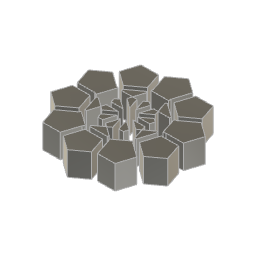
_Vent Pattern.50e8ad99-56d1-49d6-96c2-bcab84f8e137 (Autodesk Fusion 360 design; units mm, degrees)
Autodesk Fusion 360 part; units mm, degrees
note: some values were not read from the file. Chosen so that the rebuilt part matches the saved one: which bodies a step acts on.
sketch "Sketch1" plane through (0, 0, 16.5) normal (0, 0, 1) x (-1, 0, 0)
  line L0 (-58.1352, 10.5579) -> (-59.2385, 7.0968)
  line L1 (-59.2385, 7.0968) -> (-56.2877, 4.9779)
  line L2 (-56.2877, 4.9779) -> (-53.3607, 7.1296)
  line L3 (-53.3607, 7.1296) -> (-54.5025, 10.5782)
  line L4 (-54.5025, 10.5782) -> (-58.1352, 10.5579)
  line L5 (-54.5025, 10.5782) -> (-53.3607, 7.1296)
  line L6 (-53.3607, 7.1296) -> (-52.8861, 7.2867)
  line L7 (-52.8861, 7.2867) -> (-54.0279, 10.7353)
  line L8 (-54.0279, 10.7353) -> (-54.5025, 10.5782)
  line L9 (-58.1352, 10.5579) -> (-59.2385, 7.0968)
  line L10 (-59.2385, 7.0968) -> (-59.7149, 7.2486)
  line L11 (-59.7149, 7.2486) -> (-58.6116, 10.7098)
  line L12 (-58.6116, 10.7098) -> (-58.1352, 10.5579)
  line L13 (-50.6262, 13.0441) -> (-47.6754, 10.9252)
  line L14 (-47.3838, 11.3314) -> (-50.3346, 13.4502)
  line L15 (-48.7787, 7.4641) -> (-52.4114, 7.4439)
  line L16 (-54.0279, 10.7353) -> (-53.5532, 10.8925)
  line L17 (-53.5532, 10.8925) -> (-50.6262, 13.0441)
  line L18 (-53.5532, 10.8925) -> (-52.4114, 7.4439)
  line L19 (-50.6262, 13.0441) -> (-47.6754, 10.9252)
  line L20 (-52.4114, 7.4439) -> (-52.8861, 7.2867)
  line L21 (-52.8861, 7.2867) -> (-54.0279, 10.7353)
  line L22 (-50.3346, 13.4502) -> (-50.6262, 13.0441)
  line L23 (-47.6754, 10.9252) -> (-48.7787, 7.4641)
  line L24 (-47.6754, 10.9252) -> (-47.3838, 11.3314)
  line L25 (-52.4114, 7.4439) -> (-53.5532, 10.8925)
  line L26 (-45.3098, 17.8377) -> (-48.9424, 17.8175)
  line L27 (-50.043, 13.8564) -> (-47.0922, 11.7375)
  line L28 (-48.9452, 18.3175) -> (-45.3126, 18.3377)
  line L29 (-47.3838, 11.3314) -> (-50.3346, 13.4502)
  line L30 (-45.307, 17.3377) -> (-48.9397, 17.3175)
  line L31 (-50.3346, 13.4502) -> (-50.043, 13.8564)
  line L32 (-47.0922, 11.7375) -> (-47.3838, 11.3314)
  line L33 (-48.9397, 17.3175) -> (-50.043, 13.8564)
  line L34 (-48.9424, 17.8175) -> (-48.9397, 17.3175)
  line L35 (-47.1601, 23.9177) -> (-47.4562, 24.3205)
  line L36 (-50.043, 13.8564) -> (-47.0922, 11.7375)
  line L37 (-45.3098, 17.8377) -> (-48.9424, 17.8175)
  line L38 (-48.9397, 17.3175) -> (-45.307, 17.3377)
  line L39 (-45.307, 17.3377) -> (-45.3098, 17.8377)
  line L40 (-44.1652, 13.8891) -> (-45.307, 17.3377)
  line L41 (-48.9424, 17.8175) -> (-48.9452, 18.3175)
  line L42 (-47.0922, 11.7375) -> (-44.1652, 13.8891)
  line L43 (-45.3126, 18.3377) -> (-45.3098, 17.8377)
  line L44 (-54.5025, 10.5782) -> (-58.1352, 10.5579)
  line L45 (-58.1352, 10.5579) -> (-58.138, 11.0579)
  line L46 (-58.138, 11.0579) -> (-54.5053, 11.0781)
  line L47 (-54.5053, 11.0781) -> (-54.5025, 10.5782)
  line L48 (-48.9397, 17.3175) -> (-50.043, 13.8564)
  line L49 (-50.043, 13.8564) -> (-50.5193, 14.0082)
  line L50 (-50.5193, 14.0082) -> (-49.416, 17.4693)
  line L51 (-49.416, 17.4693) -> (-48.9397, 17.3175)
  line L52 (-54.5081, 11.5781) -> (-58.1407, 11.5579)
  line L53 (-58.1407, 11.5579) -> (-59.2826, 15.0065)
  line L54 (-59.2826, 15.0065) -> (-56.3556, 17.1581)
  line L55 (-56.3556, 17.1581) -> (-53.4048, 15.0393)
  line L56 (-53.4048, 15.0393) -> (-54.5081, 11.5781)
  line L57 (-52.8432, 19.74) -> (-49.8924, 17.6212)
  line L58 (-55.7702, 17.5884) -> (-52.8432, 19.74)
  line L59 (-54.6284, 14.1398) -> (-55.7702, 17.5884)
  line L60 (-50.9957, 14.1601) -> (-54.6284, 14.1398)
  line L61 (-49.8924, 17.6212) -> (-50.9957, 14.1601)
  line L62 (-50.5193, 14.0082) -> (-49.416, 17.4693)
  line L63 (-58.2127, 24.4741) -> (-54.5801, 24.4943)
  line L64 (-53.4796, 28.4555) -> (-54.5829, 24.9943)
  line L65 (-54.1065, 24.8425) -> (-54.5829, 24.9943)
  line L66 (-58.2155, 24.9741) -> (-59.3573, 28.4227)
  line L67 (-53.4796, 28.4555) -> (-53.0032, 28.3036)
  line L68 (-59.832, 28.2655) -> (-58.6902, 24.8169)
  line L69 (-54.5829, 24.9943) -> (-58.2155, 24.9741)
  line L70 (-52.5268, 28.1517) -> (-53.0032, 28.3036)
  line L71 (-51.0364, 21.4517) -> (-54.669, 21.4315)
  line L72 (-53.6301, 24.6906) -> (-50.6793, 22.5718)
  line L73 (-54.5801, 24.4943) -> (-54.5829, 24.9943)
  line L74 (-54.669, 21.4315) -> (-55.7723, 17.9704)
  line L75 (-59.3573, 28.4227) -> (-59.832, 28.2655)
  line L76 (-53.0032, 28.3036) -> (-54.1065, 24.8425)
  line L77 (-54.5829, 24.9943) -> (-53.4796, 28.4555)
  line L78 (-56.3625, 18.3941) -> (-53.4355, 20.5458)
  line L79 (-58.21, 23.9741) -> (-59.3133, 20.513)
  line L80 (-48.8942, 28.172) -> (-52.5268, 28.1517)
  line L81 (-58.6902, 24.8169) -> (-58.2155, 24.9741)
  line L82 (-53.6301, 24.6906) -> (-52.5268, 28.1517)
  line L83 (-52.5268, 28.1517) -> (-53.6301, 24.6906)
  line L84 (-58.2155, 24.9741) -> (-59.3573, 28.4227)
  line L85 (-53.4355, 20.5458) -> (-54.5773, 23.9944)
  line L86 (-58.2155, 24.9741) -> (-58.2127, 24.4741)
  line L87 (-53.0032, 28.3036) -> (-54.1065, 24.8425)
  line L88 (-54.1065, 24.8425) -> (-53.6301, 24.6906)
  line L89 (-54.5773, 23.9944) -> (-58.21, 23.9741)
  line L90 (-49.4199, 18.1603) -> (-48.9452, 18.3175)
  line L91 (-47.1601, 23.9177) -> (-44.2093, 21.7988)
  line L92 (-48.9424, 17.8175) -> (-48.9397, 17.3175)
  line L93 (-45.3098, 17.8377) -> (-48.9424, 17.8175)
  line L94 (-45.3126, 18.3377) -> (-48.9452, 18.3175)
  line L95 (-54.5829, 24.9943) -> (-58.2155, 24.9741)
  line L96 (-45.307, 17.3377) -> (-45.3098, 17.8377)
  line L97 (-48.9452, 18.3175) -> (-45.3126, 18.3377)
  line L98 (-48.9452, 18.3175) -> (-50.087, 21.7661)
  line L99 (-47.7523, 24.7234) -> (-48.8942, 28.172)
  line L100 (-50.3832, 22.1689) -> (-50.087, 21.7661)
  line L101 (-48.9397, 17.3175) -> (-45.307, 17.3377)
  line L102 (-59.3133, 20.513) -> (-56.3625, 18.3941)
  line L103 (-47.4562, 24.3205) -> (-50.3832, 22.1689)
  line L104 (-45.3098, 17.8377) -> (-48.9424, 17.8175)
  line L105 (-49.8946, 18.0031) -> (-51.0364, 21.4517)
  line L106 (-48.9452, 18.3175) -> (-50.087, 21.7661)
  line L107 (-56.4304, 30.5743) -> (-53.4796, 28.4555)
  line L108 (-50.6793, 22.5718) -> (-47.7523, 24.7234)
  line L109 (-47.4562, 24.3205) -> (-50.3832, 22.1689)
  line L110 (-50.5617, 21.6089) -> (-49.4199, 18.1603)
  line L111 (-47.1601, 23.9177) -> (-47.4562, 24.3205)
  line L112 (-50.087, 21.7661) -> (-47.1601, 23.9177)
  line L113 (-50.5617, 21.6089) -> (-49.4199, 18.1603)
  line L114 (-50.087, 21.7661) -> (-50.5617, 21.6089)
  line L115 (-50.087, 21.7661) -> (-47.1601, 23.9177)
  line L116 (-47.7523, 24.7234) -> (-47.4562, 24.3205)
  line L117 (-50.3832, 22.1689) -> (-50.6793, 22.5718)
  line L118 (-52.8215, 15.8515) -> (-49.8946, 18.0031)
  line L119 (-44.2093, 21.7988) -> (-45.3126, 18.3377)
  line L120 (-59.3573, 28.4227) -> (-56.4304, 30.5743)
  line L121 (-48.9424, 17.8175) -> (-48.9452, 18.3175)
  line L122 (-50.6793, 22.5718) -> (-47.7523, 24.7234)
  line L123 (-55.7723, 17.9704) -> (-52.8215, 15.8515)
  line L124 (-45.3126, 18.3377) -> (-45.3098, 17.8377)
  line L125 (-57.0963, 13.817) -> (-54.1455, 11.6982)
  line L126 (-53.8493, 11.2953) -> (-53.5532, 10.8925)
  line L127 (-52.3603, 17.2984) -> (-55.993, 17.2782)
  line L128 (-52.4114, 7.4439) -> (-52.8861, 7.2867)
  line L129 (-68.5088, 13.7534) -> (-65.558, 11.6346)
  line L130 (-51.2185, 13.8498) -> (-52.3603, 17.2984)
  line L131 (-53.5532, 10.8925) -> (-52.4114, 7.4439)
  line L132 (-67.4055, 17.2145) -> (-67.4083, 17.7145)
  line L133 (-67.4055, 17.2145) -> (-68.5088, 13.7534)
  line L134 (-47.3838, 11.3314) -> (-50.3346, 13.4502)
  line L135 (-50.6262, 13.0441) -> (-47.6754, 10.9252)
  line L136 (-53.5532, 10.8925) -> (-50.6262, 13.0441)
  line L137 (-54.5025, 10.5782) -> (-58.1352, 10.5579)
  line L138 (-50.3346, 13.4502) -> (-50.6262, 13.0441)
  line L139 (-65.558, 11.6346) -> (-65.2618, 11.2317)
  line L140 (-56.2877, 4.9779) -> (-53.3607, 7.1296)
  line L141 (-47.6754, 10.9252) -> (-47.3838, 11.3314)
  line L142 (-54.1455, 11.6982) -> (-51.2185, 13.8498)
  line L143 (-67.4055, 17.2145) -> (-67.4083, 17.7145)
  line L144 (-63.7728, 17.2348) -> (-63.2982, 17.392)
  line L145 (-62.631, 13.7862) -> (-63.7728, 17.2348)
  line L146 (-53.5532, 10.8925) -> (-50.6262, 13.0441)
  line L147 (-65.558, 11.6346) -> (-65.2618, 11.2317)
  line L148 (-58.5047, 11.6739) -> (-55.5777, 13.8255)
  line L149 (-50.6262, 13.0441) -> (-50.9224, 13.4469)
  line L150 (-50.6262, 13.0441) -> (-47.6754, 10.9252)
  line L151 (-50.9224, 13.4469) -> (-53.8493, 11.2953)
  line L152 (-62.0387, 12.9805) -> (-64.9657, 10.8289)
  line L153 (-58.7963, 11.2678) -> (-61.7471, 13.3866)
  line L154 (-54.0279, 10.7353) -> (-54.5025, 10.5782)
  line L155 (-54.0279, 10.7353) -> (-53.5532, 10.8925)
  line L156 (-59.2385, 7.0968) -> (-59.7149, 7.2486)
  line L157 (-55.5777, 13.8255) -> (-56.7195, 17.2741)
  line L158 (-59.0879, 10.8616) -> (-60.1912, 7.4005)
  line L159 (-60.1912, 7.4005) -> (-59.7149, 7.2486)
  line L160 (-53.3607, 7.1296) -> (-52.8861, 7.2867)
  line L161 (-52.8861, 7.2867) -> (-54.0279, 10.7353)
  line L162 (-54.5025, 10.5782) -> (-53.3607, 7.1296)
  line L163 (-53.3607, 7.1296) -> (-54.5025, 10.5782)
  line L164 (-55.993, 17.2782) -> (-57.0963, 13.817)
  line L165 (-65.6259, 23.8147) -> (-65.3342, 24.2209)
  line L166 (-65.2618, 11.2317) -> (-62.3349, 13.3833)
  line L167 (-58.049, 14.1208) -> (-61.6817, 14.1005)
  line L168 (-62.631, 13.7862) -> (-65.558, 11.6346)
  line L169 (-63.2982, 17.392) -> (-62.1563, 13.9433)
  line L170 (-63.7728, 17.2348) -> (-67.4055, 17.2145)
  line L171 (-63.7728, 17.2348) -> (-67.4055, 17.2145)
  line L172 (-67.4083, 17.7145) -> (-63.7756, 17.7348)
  line L173 (-65.2618, 11.2317) -> (-62.3349, 13.3833)
  line L174 (-67.411, 18.2145) -> (-67.4083, 17.7145)
  line L175 (-65.2618, 11.2317) -> (-62.3349, 13.3833)
  line L176 (-67.4083, 17.7145) -> (-63.7756, 17.7348)
  line L177 (-56.9457, 17.5819) -> (-58.049, 14.1208)
  line L178 (-68.5529, 21.6631) -> (-65.6259, 23.8147)
  line L179 (-55.6218, 21.7352) -> (-56.7251, 18.2741)
  line L180 (-62.0918, 22.5082) -> (-59.1648, 24.6598)
  line L181 (-60.3067, 28.1084) -> (-63.9393, 28.0881)
  line L182 (-65.2618, 11.2317) -> (-62.3349, 13.3833)
  line L183 (-62.3349, 13.3833) -> (-62.631, 13.7862)
  line L184 (-65.0426, 24.627) -> (-65.3342, 24.2209)
  line L185 (-63.7784, 18.2348) -> (-67.411, 18.2145)
  line L186 (-62.1563, 13.9433) -> (-62.631, 13.7862)
  line L187 (-61.6817, 14.1005) -> (-62.8235, 17.5491)
  line L188 (-62.6751, 21.6959) -> (-63.7784, 18.2348)
  line L189 (-62.631, 13.7862) -> (-63.7728, 17.2348)
  line L190 (-63.7756, 17.7348) -> (-63.7728, 17.2348)
  line L191 (-65.6259, 23.8147) -> (-62.6751, 21.6959)
  line L192 (-63.7784, 18.2348) -> (-67.411, 18.2145)
  line L193 (-62.3349, 13.3833) -> (-62.631, 13.7862)
  line L194 (-65.558, 11.6346) -> (-62.631, 13.7862)
  line L195 (-62.6751, 21.6959) -> (-65.6259, 23.8147)
  line L196 (-67.411, 18.2145) -> (-68.5529, 21.6631)
  line L197 (-62.631, 13.7862) -> (-65.558, 11.6346)
  line L198 (-63.7756, 17.7348) -> (-63.7784, 18.2348)
  line L199 (-63.2982, 17.392) -> (-62.1563, 13.9433)
  line L200 (-52.4114, 7.4439) -> (-53.5532, 10.8925)
  line L201 (-52.8861, 7.2867) -> (-54.0279, 10.7353)
  line L202 (-59.0879, 10.8616) -> (-60.1912, 7.4005)
  line L203 (-62.0387, 12.9805) -> (-59.0879, 10.8616)
  line L204 (-61.4555, 13.7927) -> (-58.5047, 11.6739)
  line L205 (-59.2385, 7.0968) -> (-56.2877, 4.9779)
  line L206 (-58.1352, 10.5579) -> (-59.2385, 7.0968)
  line L207 (-61.7471, 13.3866) -> (-62.0387, 12.9805)
  line L208 (-59.7149, 7.2486) -> (-58.6116, 10.7098)
  line L209 (-60.1912, 7.4005) -> (-63.8239, 7.3803)
  line L210 (-62.0387, 12.9805) -> (-59.0879, 10.8616)
  line L211 (-58.6116, 10.7098) -> (-58.1352, 10.5579)
  line L212 (-63.8239, 7.3803) -> (-64.9657, 10.8289)
  line L213 (-59.0879, 10.8616) -> (-58.7963, 11.2678)
  line L214 (-48.7787, 7.4641) -> (-52.4114, 7.4439)
  line L215 (-58.6116, 10.7098) -> (-59.0879, 10.8616)
  line L216 (-62.0387, 12.9805) -> (-64.9657, 10.8289)
  line L217 (-64.9657, 10.8289) -> (-62.0387, 12.9805)
  line L218 (-64.9657, 10.8289) -> (-65.2618, 11.2317)
  line L219 (-47.6754, 10.9252) -> (-48.7787, 7.4641)
  line L220 (-59.7149, 7.2486) -> (-58.6116, 10.7098)
  line L221 (-58.1352, 10.5579) -> (-59.2385, 7.0968)
  line L222 (-58.7963, 11.2678) -> (-61.7471, 13.3866)
  line L223 (-62.3349, 13.3833) -> (-62.0387, 12.9805)
  line L224 (-65.3342, 24.2209) -> (-62.3835, 22.102)
  line L225 (-60.3522, 17.2539) -> (-61.4555, 13.7927)
  line L226 (-59.1648, 24.6598) -> (-58.8687, 24.2569)
  line L227 (-59.1648, 24.6598) -> (-60.3067, 28.1084)
  line L228 (-59.8965, 19.7007) -> (-56.9457, 17.5819)
  line L229 (-62.0918, 22.5082) -> (-59.1648, 24.6598)
  line L230 (-64.9657, 10.8289) -> (-65.2618, 11.2317)
  line L231 (-58.8687, 24.2569) -> (-61.7957, 22.1053)
  line L232 (-60.3067, 28.1084) -> (-59.832, 28.2655)
  line L233 (-56.7195, 17.2741) -> (-60.3522, 17.2539)
  line L234 (-63.9393, 28.0881) -> (-65.0426, 24.627)
  line L235 (-58.6902, 24.8169) -> (-59.1648, 24.6598)
  line L236 (-58.5726, 23.8541) -> (-55.6218, 21.7352)
  line L237 (-62.3835, 22.102) -> (-62.6751, 21.6959)
  line L238 (-65.0426, 24.627) -> (-62.0918, 22.5082)
  line L239 (-61.7957, 22.1053) -> (-62.0918, 22.5082)
  line L240 (-62.8235, 17.5491) -> (-59.8965, 19.7007)
  line L241 (-62.3349, 13.3833) -> (-62.0387, 12.9805)
  line L242 (-62.3835, 22.102) -> (-62.0918, 22.5082)
  line L243 (-65.3342, 24.2209) -> (-62.3835, 22.102)
  line L244 (-59.832, 28.2655) -> (-58.6902, 24.8169)
  line L245 (-60.3577, 18.2538) -> (-61.4995, 21.7024)
  line L246 (-56.7251, 18.2741) -> (-60.3577, 18.2538)
  line L247 (-61.4995, 21.7024) -> (-58.5726, 23.8541)
  line L248 (-59.1648, 24.6598) -> (-60.3067, 28.1084)
  line L249 (-62.0918, 22.5082) -> (-65.0426, 24.627)
  line L250 (-58.6902, 24.8169) -> (-59.1648, 24.6598)
  line L251 (-65.0426, 24.627) -> (-62.0918, 22.5082)
  line L252 (-59.3573, 28.4227) -> (-59.832, 28.2655)
  line L253 (-58.2155, 24.9741) -> (-58.2127, 24.4741)
  line L254 (-52.8215, 15.8515) -> (-49.8946, 18.0031)
  line L255 (-62.0918, 22.5082) -> (-59.1648, 24.6598)
  line L256 (-63.9393, 28.0881) -> (-65.0426, 24.627)
  line L257 (-65.0426, 24.627) -> (-65.3342, 24.2209)
  line L258 (-60.3067, 28.1084) -> (-63.9393, 28.0881)
  line L259 (-58.2155, 24.9741) -> (-59.3573, 28.4227)
  line L260 (-65.6259, 23.8147) -> (-65.3342, 24.2209)
  line L261 (-58.2155, 24.9741) -> (-59.3573, 28.4227)
  line L262 (-60.3577, 18.2538) -> (-61.4995, 21.7024)
  line L263 (-58.2155, 24.9741) -> (-59.3573, 28.4227)
  line L264 (-58.0897, 21.4124) -> (-61.7223, 21.3922)
  line L265 (-62.3835, 22.102) -> (-62.0918, 22.5082)
  line L266 (-65.3342, 24.2209) -> (-62.3835, 22.102)
  line L267 (-65.3342, 24.2209) -> (-62.3835, 22.102)
  line L268 (-63.7784, 18.2348) -> (-67.411, 18.2145)
  line L269 (-63.7756, 17.7348) -> (-63.7784, 18.2348)
  line L270 (-60.3067, 28.1084) -> (-59.832, 28.2655)
  line L271 (-56.4304, 30.5743) -> (-53.4796, 28.4555)
  line L272 (-63.302, 18.0829) -> (-62.1987, 21.544)
  line L273 (-62.6751, 21.6959) -> (-63.7784, 18.2348)
  line L274 (-62.3835, 22.102) -> (-62.6751, 21.6959)
  line L275 (-62.3835, 22.102) -> (-62.0918, 22.5082)
  line L276 (-67.4083, 17.7145) -> (-63.7756, 17.7348)
  line L277 (-68.5529, 21.6631) -> (-65.6259, 23.8147)
  line L278 (-61.7957, 22.1053) -> (-62.0918, 22.5082)
  line L279 (-67.411, 18.2145) -> (-67.4083, 17.7145)
  line L280 (-62.6751, 21.6959) -> (-65.6259, 23.8147)
  line L281 (-62.1987, 21.544) -> (-62.6751, 21.6959)
  line L282 (-62.3835, 22.102) -> (-62.6751, 21.6959)
  line L283 (-62.6751, 21.6959) -> (-63.7784, 18.2348)
  line L284 (-63.7784, 18.2348) -> (-67.411, 18.2145)
  line L285 (-61.4995, 21.7024) -> (-58.5726, 23.8541)
  line L286 (-67.411, 18.2145) -> (-68.5529, 21.6631)
  line L287 (-61.7223, 21.3922) -> (-62.8256, 17.9311)
  line L288 (-62.6751, 21.6959) -> (-65.6259, 23.8147)
  line L289 (-63.7784, 18.2348) -> (-63.302, 18.0829)
  line L290 (-67.411, 18.2145) -> (-67.4083, 17.7145)
  line L291 (-63.302, 18.0829) -> (-62.1987, 21.544)
  line L292 (-65.6259, 23.8147) -> (-62.6751, 21.6959)
  line L293 (-53.6301, 24.6906) -> (-50.6793, 22.5718)
  line L294 (-54.2134, 23.8783) -> (-51.2626, 21.7595)
  line L295 (-51.0364, 21.4517) -> (-54.669, 21.4315)
  line L296 (-51.2626, 21.7595) -> (-52.3659, 18.2984)
  line L297 (-53.6301, 24.6906) -> (-50.6793, 22.5718)
  line L298 (-53.6301, 24.6906) -> (-50.6793, 22.5718)
  line L299 (-50.971, 22.1656) -> (-53.9217, 24.2845)
  line L300 (-48.8942, 28.172) -> (-52.5268, 28.1517)
  line L301 (-48.8942, 28.172) -> (-52.5268, 28.1517)
  line L302 (-54.5829, 24.9943) -> (-53.4796, 28.4555)
  line L303 (-57.1404, 21.7267) -> (-54.2134, 23.8783)
  line L304 (-54.5801, 24.4943) -> (-54.5829, 24.9943)
  line L305 (-54.5829, 24.9943) -> (-53.4796, 28.4555)
  line L306 (-54.1065, 24.8425) -> (-54.5829, 24.9943)
  line L307 (-53.0032, 28.3036) -> (-54.1065, 24.8425)
  line L308 (-54.1065, 24.8425) -> (-54.5829, 24.9943)
  line L309 (-56.4304, 30.5743) -> (-53.4796, 28.4555)
  line L310 (-53.0032, 28.3036) -> (-54.1065, 24.8425)
  line L311 (-53.6301, 24.6906) -> (-52.5268, 28.1517)
  line L312 (-54.1065, 24.8425) -> (-53.6301, 24.6906)
  line L313 (-52.5268, 28.1517) -> (-53.6301, 24.6906)
  line L314 (-53.4796, 28.4555) -> (-53.0032, 28.3036)
  line L315 (-52.5268, 28.1517) -> (-53.6301, 24.6906)
  line L316 (-53.0032, 28.3036) -> (-54.1065, 24.8425)
  line L317 (-53.9217, 24.2845) -> (-53.6301, 24.6906)
  line L318 (-59.3573, 28.4227) -> (-56.4304, 30.5743)
  line L319 (-56.3625, 18.3941) -> (-53.4355, 20.5458)
  line L320 (-53.4796, 28.4555) -> (-54.5829, 24.9943)
  line L321 (-54.669, 21.4315) -> (-55.7723, 17.9704)
  line L322 (-53.6301, 24.6906) -> (-52.5268, 28.1517)
  line L323 (-53.0032, 28.3036) -> (-54.1065, 24.8425)
  line L324 (-54.1065, 24.8425) -> (-53.6301, 24.6906)
  line L325 (-53.4355, 20.5458) -> (-54.5773, 23.9944)
  line L326 (-58.21, 23.9741) -> (-59.3133, 20.513)
  line L327 (-45.307, 17.3377) -> (-45.3098, 17.8377)
  line L328 (-44.1652, 13.8891) -> (-45.307, 17.3377)
  line L329 (-59.832, 28.2655) -> (-58.6902, 24.8169)
  line L330 (-58.6902, 24.8169) -> (-58.2155, 24.9741)
  line L331 (-58.8687, 24.2569) -> (-61.7957, 22.1053)
  line L332 (-56.9479, 17.9638) -> (-58.0897, 21.4124)
  line L333 (-58.6902, 24.8169) -> (-58.2155, 24.9741)
  line L334 (-59.832, 28.2655) -> (-58.6902, 24.8169)
  line L335 (-56.7251, 18.2741) -> (-60.3577, 18.2538)
  line L336 (-59.832, 28.2655) -> (-58.6902, 24.8169)
  line L337 (-65.3342, 24.2209) -> (-62.3835, 22.102)
  line L338 (-50.3346, 13.4502) -> (-50.6262, 13.0441)
  line L339 (-48.9397, 17.3175) -> (-50.043, 13.8564)
  line L340 (-54.5829, 24.9943) -> (-58.2155, 24.9741)
  line L341 (-48.9397, 17.3175) -> (-50.043, 13.8564)
  line L342 (-48.9424, 17.8175) -> (-48.9397, 17.3175)
  line L343 (-59.3133, 20.513) -> (-56.3625, 18.3941)
  line L344 (-58.8687, 24.2569) -> (-61.7957, 22.1053)
  line L345 (-65.0426, 24.627) -> (-65.3342, 24.2209)
  line L346 (-50.6262, 13.0441) -> (-47.6754, 10.9252)
  line L347 (-53.3607, 7.1296) -> (-52.8861, 7.2867)
  line L348 (-48.9424, 17.8175) -> (-48.9397, 17.3175)
  line L349 (-52.4114, 7.4439) -> (-52.8861, 7.2867)
  line L350 (-45.3098, 17.8377) -> (-48.9424, 17.8175)
  line L351 (-65.3342, 24.2209) -> (-62.3835, 22.102)
  line L352 (-50.043, 13.8564) -> (-50.5193, 14.0082)
  line L353 (-58.2155, 24.9741) -> (-59.3573, 28.4227)
  line L354 (-47.6754, 10.9252) -> (-48.7787, 7.4641)
  line L355 (-59.1648, 24.6598) -> (-58.8687, 24.2569)
  line L356 (-47.0922, 11.7375) -> (-44.1652, 13.8891)
  line L357 (-47.0922, 11.7375) -> (-47.3838, 11.3314)
  line L358 (-47.3838, 11.3314) -> (-50.3346, 13.4502)
  line L359 (-48.9397, 17.3175) -> (-45.307, 17.3377)
  line L360 (-50.6262, 13.0441) -> (-47.6754, 10.9252)
  line L361 (-50.3346, 13.4502) -> (-50.043, 13.8564)
  line L362 (-50.5193, 14.0082) -> (-49.416, 17.4693)
  line L363 (-48.7787, 7.4641) -> (-52.4114, 7.4439)
  line L364 (-62.0918, 22.5082) -> (-65.0426, 24.627)
  line L365 (-65.6259, 23.8147) -> (-65.3342, 24.2209)
  line L366 (-53.5532, 10.8925) -> (-50.6262, 13.0441)
  line L367 (-59.3573, 28.4227) -> (-59.832, 28.2655)
  line L368 (-59.1648, 24.6598) -> (-60.3067, 28.1084)
  line L369 (-62.0918, 22.5082) -> (-65.0426, 24.627)
  line L370 (-62.0918, 22.5082) -> (-59.1648, 24.6598)
  line L371 (-54.5829, 24.9943) -> (-58.2155, 24.9741)
  line L372 (-49.8924, 17.6212) -> (-50.9957, 14.1601)
  line L373 (-50.5193, 14.0082) -> (-49.416, 17.4693)
  line L374 (-58.2127, 24.4741) -> (-54.5801, 24.4943)
  line L375 (-54.5773, 23.9944) -> (-58.21, 23.9741)
  line L376 (-49.416, 17.4693) -> (-48.9397, 17.3175)
  line L377 (-54.5829, 24.9943) -> (-58.2155, 24.9741)
  line L378 (-58.5726, 23.8541) -> (-55.6218, 21.7352)
  line L379 (-48.9424, 17.8175) -> (-48.9452, 18.3175)
  line L380 (-59.1648, 24.6598) -> (-60.3067, 28.1084)
  line L381 (-53.5532, 10.8925) -> (-52.4114, 7.4439)
  line L382 (-52.4114, 7.4439) -> (-53.5532, 10.8925)
  line L383 (-45.307, 17.3377) -> (-45.3098, 17.8377)
  line L384 (-47.0922, 11.7375) -> (-47.3838, 11.3314)
  line L385 (-45.3098, 17.8377) -> (-48.9424, 17.8175)
  line L386 (-47.6754, 10.9252) -> (-47.3838, 11.3314)
  line L387 (-47.3838, 11.3314) -> (-50.3346, 13.4502)
  line L388 (-58.1352, 10.5579) -> (-59.2385, 7.0968)
  line L389 (-54.5081, 11.5781) -> (-58.1407, 11.5579)
  line L390 (-59.2385, 7.0968) -> (-56.2877, 4.9779)
  line L391 (-50.043, 13.8564) -> (-47.0922, 11.7375)
  line L392 (-59.2826, 15.0065) -> (-56.3556, 17.1581)
  line L393 (-62.3349, 13.3833) -> (-62.631, 13.7862)
  line L394 (-45.3098, 17.8377) -> (-48.9424, 17.8175)
  line L395 (-58.1352, 10.5579) -> (-58.138, 11.0579)
  line L396 (-60.3522, 17.2539) -> (-61.4555, 13.7927)
  line L397 (-64.9657, 10.8289) -> (-65.2618, 11.2317)
  line L398 (-59.2385, 7.0968) -> (-59.7149, 7.2486)
  line L399 (-68.5088, 13.7534) -> (-65.558, 11.6346)
  line L400 (-54.6284, 14.1398) -> (-55.7702, 17.5884)
  line L401 (-54.5025, 10.5782) -> (-58.1352, 10.5579)
  line L402 (-54.0279, 10.7353) -> (-54.5025, 10.5782)
  line L403 (-63.7728, 17.2348) -> (-67.4055, 17.2145)
  line L404 (-58.1352, 10.5579) -> (-59.2385, 7.0968)
  line L405 (-62.3349, 13.3833) -> (-62.0387, 12.9805)
  line L406 (-63.8239, 7.3803) -> (-64.9657, 10.8289)
  line L407 (-61.7471, 13.3866) -> (-62.0387, 12.9805)
  line L408 (-55.5777, 13.8255) -> (-56.7195, 17.2741)
  line L409 (-58.6116, 10.7098) -> (-58.1352, 10.5579)
  line L410 (-58.1407, 11.5579) -> (-59.2826, 15.0065)
  line L411 (-63.7728, 17.2348) -> (-67.4055, 17.2145)
  line L412 (-67.4055, 17.2145) -> (-68.5088, 13.7534)
  line L413 (-65.558, 11.6346) -> (-65.2618, 11.2317)
  line L414 (-62.0387, 12.9805) -> (-64.9657, 10.8289)
  line L415 (-65.2618, 11.2317) -> (-62.3349, 13.3833)
  line L416 (-62.631, 13.7862) -> (-63.7728, 17.2348)
  line L417 (-64.9657, 10.8289) -> (-62.0387, 12.9805)
  line L418 (-58.138, 11.0579) -> (-54.5053, 11.0781)
  line L419 (-50.043, 13.8564) -> (-47.0922, 11.7375)
  line L420 (-45.307, 17.3377) -> (-48.9397, 17.3175)
  line L421 (-59.7149, 7.2486) -> (-58.6116, 10.7098)
  line L422 (-58.6116, 10.7098) -> (-59.0879, 10.8616)
  line L423 (-54.5025, 10.5782) -> (-58.1352, 10.5579)
  line L424 (-48.9397, 17.3175) -> (-45.307, 17.3377)
  line L425 (-54.5053, 11.0781) -> (-54.5025, 10.5782)
  line L426 (-45.3098, 17.8377) -> (-48.9424, 17.8175)
  line L427 (-58.5047, 11.6739) -> (-55.5777, 13.8255)
  line L428 (-59.0879, 10.8616) -> (-58.7963, 11.2678)
  line L429 (-59.7149, 7.2486) -> (-58.6116, 10.7098)
  line L430 (-48.9452, 18.3175) -> (-45.3126, 18.3377)
  line L431 (-50.5617, 21.6089) -> (-49.4199, 18.1603)
  line L432 (-47.7523, 24.7234) -> (-47.4562, 24.3205)
  line L433 (-59.3573, 28.4227) -> (-56.4304, 30.5743)
  line L434 (-50.6793, 22.5718) -> (-47.7523, 24.7234)
  line L435 (-47.4562, 24.3205) -> (-50.3832, 22.1689)
  line L436 (-48.9452, 18.3175) -> (-50.087, 21.7661)
  line L437 (-47.7523, 24.7234) -> (-47.4562, 24.3205)
  line L438 (-50.087, 21.7661) -> (-50.5617, 21.6089)
  line L439 (-50.6793, 22.5718) -> (-47.7523, 24.7234)
  line L440 (-47.7523, 24.7234) -> (-48.8942, 28.172)
  line L441 (-50.5617, 21.6089) -> (-49.4199, 18.1603)
  line L442 (-47.4562, 24.3205) -> (-50.3832, 22.1689)
  line L443 (-47.4562, 24.3205) -> (-50.3832, 22.1689)
  line L444 (-50.6793, 22.5718) -> (-47.7523, 24.7234)
  line L445 (-47.1601, 23.9177) -> (-47.4562, 24.3205)
  line L446 (-48.9452, 18.3175) -> (-45.3126, 18.3377)
  line L447 (-50.6793, 22.5718) -> (-50.971, 22.1656)
  line L448 (-50.3832, 22.1689) -> (-50.6793, 22.5718)
  line L449 (-44.2093, 21.7988) -> (-45.3126, 18.3377)
  line L450 (-50.6793, 22.5718) -> (-47.7523, 24.7234)
  line L451 (-49.4199, 18.1603) -> (-48.9452, 18.3175)
  line L452 (-50.087, 21.7661) -> (-47.1601, 23.9177)
  line L453 (-48.9452, 18.3175) -> (-50.087, 21.7661)
  line L454 (-50.3832, 22.1689) -> (-50.087, 21.7661)
  line L455 (-55.6218, 21.7352) -> (-56.7251, 18.2741)
  line L456 (-52.5268, 28.1517) -> (-53.0032, 28.3036)
  line L457 (-49.8946, 18.0031) -> (-51.0364, 21.4517)
  line L458 (-47.7523, 24.7234) -> (-48.8942, 28.172)
  line L459 (-53.4796, 28.4555) -> (-53.0032, 28.3036)
  line L460 (-50.3832, 22.1689) -> (-50.6793, 22.5718)
  line L461 (-52.3659, 18.2984) -> (-55.9985, 18.2781)
  line L462 (-47.1601, 23.9177) -> (-44.2093, 21.7988)
  line L463 (-50.087, 21.7661) -> (-47.1601, 23.9177)
  line L464 (-53.4796, 28.4555) -> (-54.5829, 24.9943)
  line L465 (-45.3126, 18.3377) -> (-48.9452, 18.3175)
  line L466 (-55.9985, 18.2781) -> (-57.1404, 21.7267)
  line L467 (-52.5268, 28.1517) -> (-53.0032, 28.3036)
  line L468 (-62.631, 13.7862) -> (-65.558, 11.6346)
  line L469 (-65.2618, 11.2317) -> (-62.3349, 13.3833)
  line L470 (-56.2877, 4.9779) -> (-53.3607, 7.1296)
  line L471 (-54.0279, 10.7353) -> (-53.5532, 10.8925)
  line L472 (-55.7723, 17.9704) -> (-52.8215, 15.8515)
  line L473 (-58.7963, 11.2678) -> (-61.7471, 13.3866)
  line L474 (-59.8748, 15.8122) -> (-56.9479, 17.9638)
  line L475 (-54.5025, 10.5782) -> (-53.3607, 7.1296)
  line L476 (-45.3126, 18.3377) -> (-45.3098, 17.8377)
  line L477 (-53.3607, 7.1296) -> (-54.5025, 10.5782)
  line L478 (-52.8861, 7.2867) -> (-54.0279, 10.7353)
  line L479 (-61.4555, 13.7927) -> (-58.5047, 11.6739)
  line L480 (-52.8432, 19.74) -> (-49.8924, 17.6212)
  line L481 (-59.0879, 10.8616) -> (-60.1912, 7.4005)
  line L482 (-50.9957, 14.1601) -> (-54.6284, 14.1398)
  line L483 (-62.8256, 17.9311) -> (-59.8748, 15.8122)
  line L484 (-65.558, 11.6346) -> (-62.631, 13.7862)
  line L485 (-62.0387, 12.9805) -> (-59.0879, 10.8616)
  line L486 (-56.7195, 17.2741) -> (-60.3522, 17.2539)
  line L487 (-60.1912, 7.4005) -> (-63.8239, 7.3803)
  line L488 (-59.0879, 10.8616) -> (-60.1912, 7.4005)
  line L489 (-52.8861, 7.2867) -> (-54.0279, 10.7353)
  line L490 (-67.4055, 17.2145) -> (-67.4083, 17.7145)
  line L491 (-63.7756, 17.7348) -> (-63.7728, 17.2348)
  line L492 (-56.3556, 17.1581) -> (-53.4048, 15.0393)
  line L493 (-45.3126, 18.3377) -> (-45.3098, 17.8377)
  line L494 (-60.1912, 7.4005) -> (-59.7149, 7.2486)
  line L495 (-53.4048, 15.0393) -> (-54.5081, 11.5781)
  line L496 (-62.0387, 12.9805) -> (-59.0879, 10.8616)
  line L497 (-48.9424, 17.8175) -> (-48.9452, 18.3175)
  line L498 (-55.7702, 17.5884) -> (-52.8432, 19.74)
  point P0 (-56.3049, 8.0681)
  point P1 (-50.609, 9.954)
  point P2 (-47.1094, 14.8276)
  point P3 (-50.6965, 25.6619)
  point P4 (-47.1428, 20.8275)
  point P5 (-56.4131, 27.4842)
  point P6 (-62.1091, 25.5983)
  point P7 (-65.6087, 20.7246)
  point P8 (-62.0215, 9.8903)
  point P9 (-56.3049, 8.0681)
  point P10 (-50.609, 9.954)
  point P11 (-65.5752, 14.7247)
  point P12 (-65.6087, 20.7246)
  point P13 (-56.4131, 27.4842)
  point P14 (-62.1091, 25.5983)
  point P15 (-56.4131, 27.4842)
  point P16 (-50.6965, 25.6619)
  point P17 (-50.6965, 25.6619)
  point P18 (-47.1428, 20.8275)
  point P19 (-50.609, 9.954)
  point P20 (-47.1094, 14.8276)
  point P21 (-62.0215, 9.8903)
  point P22 (-65.5752, 14.7247)
  point P23 (-56.3049, 8.0681)
  dimension "d1" = 2.5
  dimension "d2" = 0.5
  dimension "d3" = 0.5
  dimension "d4" = 0.5
  dimension "d5" = 0.5
  constraint perpendicular L5 L6
  constraint parallel L5 L7
  constraint parallel L6 L8
  constraint perpendicular L9 L10
  constraint parallel L9 L11
  constraint parallel L10 L12
  constraint symmetric L0.start L7 L13.start
  constraint symmetric L0.end L7 L13.end
  constraint symmetric L1.end L7 L15.start
  constraint symmetric L2.end L7 L15.end
  constraint symmetric L3.end L7 L16.end
  constraint symmetric P23 L7 P19
  constraint symmetric L6.end L7 L20.end
  constraint symmetric L8.start L7 L16.start
  constraint symmetric L7 L10.end L14.start
  constraint symmetric L7 L11.end L14.end
  constraint symmetric L0.end L14 L35.start
  constraint symmetric L2.end L14 L28.end
  constraint symmetric L3.end L14 L28.start
  constraint symmetric L6.end L14 L26.start
  constraint symmetric L7.end L14 L26.end
  constraint symmetric L10.end L14 L35.end
  constraint symmetric P19 L14 P20
  constraint symmetric L15.end L14 L30.start
  constraint symmetric L16.end L14 L30.end
  constraint symmetric L13.end L14 L27.end
  constraint symmetric L22.start L14 L29.end
  constraint symmetric L24.end L14 L29.start
  constraint symmetric L13.start L14 L27.start
  constraint symmetric L14 L15.start L40.start
  constraint perpendicular L44 L45
  constraint parallel L44 L46
  constraint parallel L45 L47
  constraint perpendicular L48 L49
  constraint parallel L48 L50
  constraint parallel L49 L51
  constraint symmetric L0.start L46 L52.end
  constraint symmetric L0.end L46 L53.end
  constraint symmetric L1.end L46 L54.end
  constraint symmetric L2.end L46 L55.end
  constraint symmetric L3.end L46 L52.start
  constraint symmetric L30.start L50 L57.start
  constraint symmetric L30.end L50 L57.end
  constraint symmetric L27.start L50 L60.start
  constraint symmetric L40.start L50 L58.start
  constraint symmetric L27.end L50 L59.start
  constraint symmetric L49.end L50 L62.start
  constraint symmetric L51.start L50 L62.end
  constraint symmetric L0.start L26 L66.start
  constraint symmetric L0.end L26 L66.end
  constraint symmetric L1.end L26 L107.start
  constraint symmetric L2.end L26 L64.start
  constraint symmetric L3.end L26 L64.end
  constraint symmetric P23 L26 P15
  constraint symmetric L6.end L26 L67.end
  constraint symmetric L7.end L26 L65.start
  constraint symmetric L10.end L26 L68.start
  constraint symmetric L11.end L26 L68.end
  constraint symmetric P19 L26 P17
  constraint symmetric L15.end L26 L70.start
  constraint symmetric L16.end L26 L72.start
  constraint symmetric L13.end L26 L99.start
  constraint symmetric L14.end L26 L100.start
  constraint symmetric L14.start L26 L35.end
  constraint symmetric L13.start L26 L72.end
  constraint symmetric L15.start L26 L80.start
  constraint symmetric L28.end L26 L30.start
  constraint symmetric P20 L26 P18
  constraint symmetric L28.start L26 L30.end
  constraint symmetric L34.start L26 L37.end
  constraint symmetric L30.start L26 L28.end
  constraint symmetric L30.end L26 L28.start
  constraint symmetric L27.start L26 L98.end
  constraint symmetric L40.start L26 L91.end
  constraint symmetric L27.end L26 L35.start
  constraint symmetric L37.start L26 L39.end
  constraint symmetric L26 L45.end L63.start
  constraint symmetric L26 L46.end L63.end
  constraint symmetric L26 L49.end L110.start
  constraint symmetric L26 L50.end L90.start
  constraint symmetric L26 L52.start L85.end
  constraint symmetric L26 L52.end L79.start
  constraint symmetric L26 L53.end L79.end
  constraint symmetric L26 L54.end L78.start
  constraint symmetric L26 L55.end L78.end
  constraint symmetric L26 L57.start L118.start
  constraint symmetric L26 L57.end L105.start
  constraint symmetric L26 L58.start L74.end
  constraint symmetric L26 L59.start L71.end
  constraint symmetric L26 L60.start L71.start
  constraint symmetric L0.start L68 L13.start
  constraint symmetric L0.end L68 L13.end
  constraint symmetric L1.end L68 L15.start
  constraint symmetric L2.end L68 L15.end
  constraint symmetric L3.end L68 L16.end
  constraint symmetric P23 L68 P19
  constraint symmetric L6.end L68 L7.start
  constraint symmetric L7.end L68 L8.start
  constraint symmetric L10.end L68 L14.start
  constraint symmetric L11.end L68 L14.end
  constraint symmetric P19 L68 P23
  constraint symmetric L15.end L68 L2.end
  constraint symmetric L16.end L68 L3.end
  constraint symmetric L13.end L68 L0.end
  constraint symmetric L14.end L68 L11.end
  constraint symmetric L14.start L68 L10.end
  constraint symmetric L13.start L68 L0.start
  constraint symmetric L15.start L68 L1.end
  constraint symmetric L28.end L68 L129.end
  constraint symmetric P20 L68 P21
  constraint symmetric L28.start L68 L145.start
  constraint symmetric L35.start L68 L132.start
  constraint symmetric L35.end L68 L132.end
  constraint symmetric L26.end L68 L166.end
  constraint symmetric L30.start L68 L152.end
  constraint symmetric L30.end L68 L152.start
  constraint symmetric L27.start L68 L158.start
  constraint symmetric L40.start L68 L209.end
  constraint symmetric L27.end L68 L158.end
  constraint symmetric L26.start L68 L139.end
  constraint symmetric L45.end L68 L149.end
  constraint symmetric L46.end L68 L126.start
  constraint symmetric L49.end L68 L153.start
  constraint symmetric L50.end L68 L153.end
  constraint symmetric L52.start L68 L125.end
  constraint symmetric L52.end L68 L130.start
  constraint symmetric L53.end L68 L127.start
  constraint symmetric L54.end L68 L127.end
  constraint symmetric L55.end L68 L125.start
  constraint symmetric L57.start L68 L225.start
  constraint symmetric L57.end L68 L204.start
  constraint symmetric L58.start L68 L157.end
  constraint symmetric L59.start L68 L148.end
  constraint symmetric L60.start L68 L148.start
  constraint symmetric L65.start L68 L224.end
  constraint symmetric L63.start L68 L226.end
  constraint symmetric L75.end L68 L232.end
  constraint symmetric L81.start L68 L235.start
  constraint symmetric L72.start L68 L188.start
  constraint symmetric L67.end L68 L165.end
  constraint symmetric L70.start L68 L165.start
  constraint symmetric L85.end L68 L245.end
  constraint symmetric L64.start L68 L184.start
  constraint symmetric L74.end L68 L177.start
  constraint symmetric L107.start L68 L181.end
  constraint symmetric L118.start L68 L167.start
  constraint symmetric L79.end L68 L179.start
  constraint symmetric L64.end L68 L180.start
  constraint symmetric L78.end L68 L245.start
  constraint symmetric L78.start L68 L179.end
  constraint symmetric L79.start L68 L236.start
  constraint symmetric L63.end L68 L231.end
  constraint symmetric L71.end L68 L228.start
  constraint symmetric L72.end L68 L185.start
  constraint symmetric L66.end L68 L181.start
  constraint symmetric L105.start L68 L167.end
  constraint symmetric L98.end L68 L144.start
  constraint symmetric L99.start L68 L174.start
  constraint symmetric L71.start L68 L187.end
  constraint symmetric L110.start L68 L144.end
  constraint symmetric L100.start L68 L172.end
  constraint symmetric P17 L68 P12
  constraint symmetric L90.start L68 L169.end
  constraint symmetric L91.end L68 L129.start
  constraint symmetric L80.start L68 L178.start
  constraint symmetric P18 L68 P22
  constraint symmetric P15 L68 P14
  constraint symmetric L66.start L68 L180.end
  constraint symmetric L0.start L172 L66.start
  constraint symmetric L0.end L172 L66.end
  constraint symmetric L1.end L172 L107.start
  constraint symmetric L2.end L172 L64.start
  constraint symmetric L3.end L172 L64.end
  constraint symmetric P23 L172 P15
  constraint symmetric L6.end L172 L67.end
  constraint symmetric L7.end L172 L65.start
  constraint symmetric L10.end L172 L68.start
  constraint symmetric L11.end L172 L68.end
  constraint symmetric P19 L172 P17
  constraint symmetric L15.end L172 L70.start
  constraint symmetric L16.end L172 L72.start
  constraint symmetric L13.end L172 L99.start
  constraint symmetric L14.end L172 L100.start
  constraint symmetric L14.start L172 L35.end
  constraint symmetric L13.start L172 L72.end
  constraint symmetric L15.start L172 L80.start
  constraint symmetric L28.end L172 L30.start
  constraint symmetric P20 L172 P18
  constraint symmetric L28.start L172 L30.end
  constraint symmetric L35.start L172 L27.end
  constraint symmetric L35.end L172 L14.start
  constraint symmetric L26.end L172 L34.start
  constraint symmetric L30.start L172 L28.end
  constraint symmetric L30.end L172 L28.start
  constraint symmetric L27.start L172 L98.end
  constraint symmetric L40.start L172 L91.end
  constraint symmetric L27.end L172 L35.start
  constraint symmetric L26.start L172 L37.start
  constraint symmetric L45.end L172 L63.start
  constraint symmetric L46.end L172 L63.end
  constraint symmetric L49.end L172 L110.start
  constraint symmetric L50.end L172 L90.start
  constraint symmetric L52.start L172 L85.end
  constraint symmetric L52.end L172 L79.start
  constraint symmetric L53.end L172 L79.end
  constraint symmetric L54.end L172 L78.start
  constraint symmetric L55.end L172 L78.end
  constraint symmetric L57.start L172 L118.start
  constraint symmetric L57.end L172 L105.start
  constraint symmetric L58.start L172 L74.end
  constraint symmetric L59.start L172 L71.end
  constraint symmetric L60.start L172 L71.start
  constraint symmetric L65.start L172 L7.end
  constraint symmetric L63.start L172 L45.end
  constraint symmetric L68.start L172 L10.end
  constraint symmetric L68.end L172 L11.end
  constraint symmetric L72.start L172 L16.end
  constraint symmetric L67.end L172 L6.end
  constraint symmetric L70.start L172 L15.end
  constraint symmetric L85.end L172 L52.start
  constraint symmetric L64.start L172 L2.end
  constraint symmetric L74.end L172 L58.start
  constraint symmetric L107.start L172 L1.end
  constraint symmetric L118.start L172 L57.start
  constraint symmetric L79.end L172 L53.end
  constraint symmetric L64.end L172 L3.end
  constraint symmetric L78.end L172 L55.end
  constraint symmetric L78.start L172 L54.end
  constraint symmetric L79.start L172 L52.end
  constraint symmetric L63.end L172 L46.end
  constraint symmetric L71.end L172 L59.start
  constraint symmetric L72.end L172 L13.start
  constraint symmetric L66.end L172 L0.end
  constraint symmetric L105.start L172 L57.end
  constraint symmetric L98.end L172 L27.start
  constraint symmetric L99.start L172 L13.end
  constraint symmetric L71.start L172 L60.start
  constraint symmetric L110.start L172 L49.end
  constraint symmetric L100.start L172 L14.end
  constraint symmetric P17 L172 P19
  constraint symmetric L90.start L172 L50.end
  constraint symmetric L91.end L172 L40.start
  constraint symmetric L80.start L172 L15.start
  constraint symmetric P18 L172 P20
  constraint symmetric P15 L172 P23
  constraint symmetric L66.start L172 L0.start
  constraint symmetric L125.start L172 L303.start
  constraint symmetric L177.start L172 L332.start
  constraint symmetric L180.end L172 L158.start
  constraint symmetric L176.end L172 L190.start
  constraint symmetric L132.end L172 L143.end
  constraint symmetric L174.start L172 L132.start
  constraint symmetric L127.start L172 L296.end
  constraint symmetric L127.end L172 L461.end
  constraint symmetric L167.start L172 L264.start
  constraint symmetric L178.start L172 L129.start
  constraint symmetric L187.end L172 L287.end
  constraint symmetric L144.start L172 L185.start
  constraint symmetric L181.start L172 L158.end
  constraint symmetric L144.end L172 L272.start
  constraint symmetric L148.end L172 L179.start
  constraint symmetric L129.start L172 L178.start
  constraint symmetric L179.end L172 L157.end
  constraint symmetric L149.end L172 L299.start
  constraint symmetric L130.start L172 L294.end
  constraint symmetric L132.start L172 L174.start
  constraint symmetric L157.end L172 L179.end
  constraint symmetric L185.start L172 L144.start
  constraint symmetric L126.start L172 L299.end
  constraint symmetric L125.end L172 L294.start
  constraint symmetric L169.end L172 L272.end
  constraint symmetric L166.end L172 L224.end
  constraint symmetric L139.end L172 L165.end
  constraint symmetric L129.end L172 L165.start
  constraint symmetric L152.start L172 L180.start
  constraint symmetric P14 L172 P21
  constraint symmetric L152.end L172 L184.start
  constraint symmetric P12 L172 P22
  constraint symmetric L188.start L172 L145.start
  constraint symmetric L165.start L172 L129.end
  constraint symmetric L165.end L172 L139.end
  constraint symmetric L224.end L172 L166.end
  constraint symmetric L184.start L172 L152.end
  constraint symmetric L228.start L172 L474.start
  constraint symmetric L226.end L172 L153.start
  constraint symmetric L245.end L172 L204.start
  constraint symmetric L180.start L172 L152.start
  constraint symmetric L179.start L172 L148.end
  constraint symmetric L181.end L172 L209.end
  constraint symmetric L231.end L172 L153.end
  constraint symmetric L225.start L172 L245.start
  constraint symmetric L245.start L172 L225.start
  constraint symmetric L236.start L172 L148.start
  constraint symmetric L158.start L172 L180.end
  constraint symmetric L145.start L172 L188.start
  constraint symmetric L167.end L172 L264.end
  constraint symmetric L153.start L172 L226.end
  constraint symmetric L158.end L172 L181.start
  constraint symmetric P21 L172 P14
  constraint symmetric L204.start L172 L245.end
  constraint symmetric L148.start L172 L236.start
  constraint symmetric L209.end L172 L181.end
  constraint symmetric L153.end L172 L231.end
  constraint symmetric P22 L172 P12
  measures "d1" distance of P23 L4
  measures "d2" distance of L3.end L7.end
  measures "d3" distance of L0.start L11.end
  measures "d4" distance of L3.end L46.end
  measures "d5" distance of L30.end L50.end
extrude "Extrude1" add sketch "Sketch1" along normal blind 3 contours L0 L1 L2 L3 L4 L5 L9 L44 L137 L140 L162 L163 L205 L206 L221 L388 L390 L401 L404 L423 L470 L475 L477 | L4 L44 L45 L46 L47 L137 L395 L401 L418 L423 L425 | L152 L158 L202 L203 L209 L210 L212 L216 L217 L406 L414 L417 L481 L485 L487 L488 L496 | L13 L15 L17 L18 L19 L23 L25 L131 L135 L136 L146 L150 L200 L214 L219 L346 L354 L360 L363 L366 L381 L382 | L129 L133 L145 L168 L170 L171 L189 L194 L197 L399 L403 L411 L412 L416 L468 L484 | L144 L145 L169 L186 L189 L199 L416 | L27 L30 L33 L36 L38 L40 L42 L48 L101 L328 L339 L341 L356 L359 L391 L419 L420 L424 | L33 L48 L49 L50 L51 L62 L339 L341 L352 L362 L373 L376 | L178 L185 L188 L191 L192 L195 L196 L268 L273 L277 L280 L283 L284 L286 L288 L292 | L28 L91 L94 L97 L98 L106 L112 L115 L119 L430 L436 L446 L449 L452 L453 L462 L463 L465 | L180 L181 L227 L229 L234 L238 L248 L249 L251 L255 L256 L258 L364 L368 L369 L370 L380 | L180 L226 L229 L231 L239 L255 L278 L331 L344 L355 L370 | L72 L293 L297 L298 L299 L317 L447 | L72 L80 L82 L83 L99 L108 L122 L293 L297 L298 L300 L301 L311 L313 L315 L322 L434 L439 L440 L444 L450 L458 | L64 L66 L69 L77 L84 L95 L107 L120 L259 L261 L263 L271 L302 L305 L309 L318 L320 L340 L353 L371 L377 L433 L464 | L56 L60 L125 L130 L142 L482 L495 | L53 L148 L167 L204 L225 L396 L410 L427 L479 | L55 L56 L59 L60 L400 L482 L492 L495 | L125 L148 L157 L164 L408 L427 | L53 L54 L167 L177 L392 L410 | L118 L123 L127 L130 L254 L472 | L225 L233 L396 L474 L483 L486 | L57 L71 L105 L118 L254 L295 L296 L457 L480 | L240 L245 L262 L264 L287 L483 | L57 L58 L296 L461 L480 L498 | L228 L240 L245 L246 L262 L335 | L71 L74 L78 L85 L295 L319 L321 L325 | L79 L102 L264 L326 L332 L343 | L79 L85 L89 L236 L303 L325 L326 L375 L378 | L179 L236 L303 L378 L455 L466 makes body 3 at (55.7882, -23.9876, 17.5) makes body 3 at (55.8705, -20.9549, 17.5) makes body 9 at (62.0901, -20.2385, 17.5) makes body 9 at (58.7197, -18.263, 17.5) makes body 2 at (60.4719, -13.0865, 18.5) makes body 2 at (58.6226, -15.4916, 17.5) makes body 10 at (53.1698, -12.4154, 17.5) makes body 10 at (54.7354, -15.9947, 17.5) makes body 1 at (50.2752, -19.1527, 17.5) makes body 1 at (54.1631, -18.7698, 17.5) makes body 18 at (56.7902, -27.9971, 16.5) makes body 6 at (51.3031, -25.8553, 16.5) makes body 5 at (47.1393, -20.1909, 16.5) makes body 17 at (47.1129, -15.4642, 16.5) makes body 19 at (51.2133, -9.7539, 16.5) makes body 7 at (55.7006, -8.2682, 16.5) makes body 4 at (62.3986, -10.4033, 16.5) makes body 16 at (65.1982, -14.2118, 16.5) makes body 20 at (65.2373, -21.2417, 16.5) makes body 8 at (62.4804, -25.0812, 16.5) makes body 15 at (54.7553, -19.5755, 17.5) makes body 11 at (58.648, -20.0353, 17.5) makes body 14 at (59.2149, -16.2973, 17.5) makes body 12 at (56.5988, -15.3778, 17.5) makes body 13 at (54.1521, -16.807, 17.5)
extrude "Extrude2" add 25 faces at (62.3986, -10.4033, 19.5) (58.2115, -15.1964, 19.5) (54.478, -15.2172, 19.5) (56.3413, -14.6002, 19.5) (59.6492, -13.1941, 19.5) (62.4804, -25.0812, 19.5) (56.3767, -20.952, 19.5) (54.5066, -20.3559, 19.5) (59.374, -16.7779, 19.5) (56.3905, -23.417, 19.5) (58.2401, -20.3351, 19.5) (51.0039, -19.5492, 19.5) (51.2133, -9.7539, 19.5) (61.7336, -19.4894, 19.5) (59.385, -18.7407, 19.5) (53.344, -18.7744, 19.5) (55.7006, -8.2682, 19.5) (53.0179, -13.231, 19.5) (51.3031, -25.8553, 19.5) (56.7902, -27.9971, 19.5) (47.1129, -15.4642, 19.5) (53.3331, -16.8116, 19.5) (47.1393, -20.1909, 19.5) (65.1982, -14.2118, 19.5) (65.2373, -21.2417, 19.5) along direction (0, 0, 1) blind 2 on bodies 1 2 3 4 5 6 7 8 9 10 11 12 13 14 15 16 17 18 19 20 bodies 4 1 2 3 5 6 7 8 9 10 11 12 13 14 15 16 17 18 19 20
